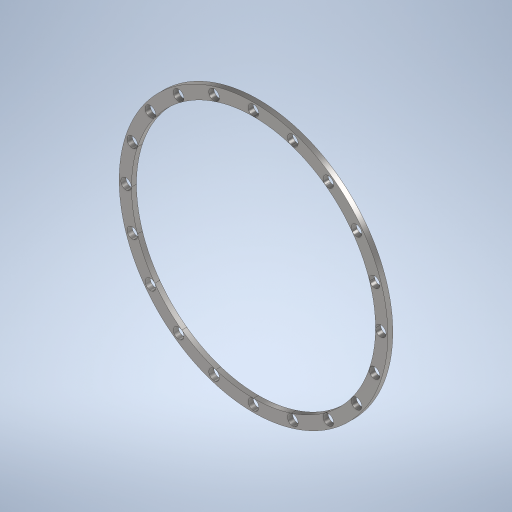
# Autodesk Inventor part: bracket 1
Saved by Autodesk Inventor 2023 (Build 270158000, 158)
## iProperties
Created: 2022-07-21
Part Number: bracket 1
Material: Stainless Steel
Document SubType Name: Modeling
Designer: station
Density: 8 g/cm^3
Appearance: Semi-Polished
Mass: 114.58 g
Surface Area: 134.314 cm^2
Volume: 14.3225 cm^3
Author: station
Autodesk Inventor part; units mm, degrees
ref_plane "YZ Plane" through (0, 0, 0) normal (1, 0, 0) x (0, 1, 0)
ref_plane "XZ Plane" through (0, 0, 0) normal (0, 1, 0) x (-1, 0, 0)
ref_plane "XY Plane" through (0, 0, 0) normal (0, 0, 1) x (1, 0, 0)
sketch "Sketch1" plane through (0, 0, 0) normal (0, 0, 1) x (1, 0, 0)
  point P0 (0, 0)
sketch "Sketch2" plane through (0, 0, 0) normal (0, 0, 1) x (1, 0, 0)
  circle A0 centre (0, 0) radius 73.505
  circle A1 centre (0, 0) radius 80.905
  line L0 (0, 0) -> (0, 267.2238)
  line L1 (0, 73.505) -> (0, 76.705)
  circle A2 centre (0, 76.705) radius 3.2
  circle A3 centre (-23.7031, 72.9508) radius 3.2
  circle A4 centre (-45.0861, 62.0556) radius 3.2
  circle A5 centre (-62.0556, 45.0861) radius 3.2
  circle A6 centre (-72.9508, 23.7031) radius 3.2
  circle A7 centre (-76.705, 0) radius 3.2
  circle A8 centre (-72.9508, -23.7031) radius 3.2
  circle A9 centre (-62.0556, -45.0861) radius 3.2
  circle A10 centre (-45.0861, -62.0556) radius 3.2
  circle A11 centre (-23.7031, -72.9508) radius 3.2
  circle A12 centre (0, -76.705) radius 3.2
  circle A13 centre (23.7031, -72.9508) radius 3.2
  circle A14 centre (45.0861, -62.0556) radius 3.2
  circle A15 centre (62.0556, -45.0861) radius 3.2
  circle A16 centre (72.9508, -23.7031) radius 3.2
  circle A17 centre (76.705, 0) radius 3.2
  circle A18 centre (72.9508, 23.7031) radius 3.2
  circle A19 centre (62.0556, 45.0861) radius 3.2
  circle A20 centre (45.0861, 62.0556) radius 3.2
  circle A21 centre (23.7031, 72.9508) radius 3.2
  point P0 (0, 73.505)
  point P1 (22.7143, 69.9074)
  point P2 (43.2052, 59.4668)
  point P3 (59.4668, 43.2052)
  point P4 (69.9074, 22.7143)
  point P5 (73.505, 0)
  point P6 (69.9074, -22.7143)
  point P7 (59.4668, -43.2052)
  point P8 (43.2052, -59.4668)
  point P9 (22.7143, -69.9074)
  point P10 (0, -73.505)
  point P11 (-22.7143, -69.9074)
  point P12 (-43.2052, -59.4668)
  point P13 (-59.4668, -43.2052)
  point P14 (-69.9074, -22.7143)
  point P15 (-73.505, 0)
  point P16 (-69.9074, 22.7143)
  point P17 (-59.4668, 43.2052)
  point P18 (-43.2052, 59.4668)
  point P19 (-22.7143, 69.9074)
  dimension "d0" = 147.01
  dimension "d1" = 161.81
  dimension "d3" = 3.2
  dimension "d4" = 6.4
  dimension "d19" = 360
  constraints: 21 centre point, 4 end point, 3 coincident, 2 point on line, 1 vertical, 44 other
  measures "d1" diameter of A1
  measures "d3" distance of L1.start L1.end
  measures "d4" diameter of A2
extrude "Extrusion3" add sketch "Sketch2" along normal blind 3
body "Solid2"
